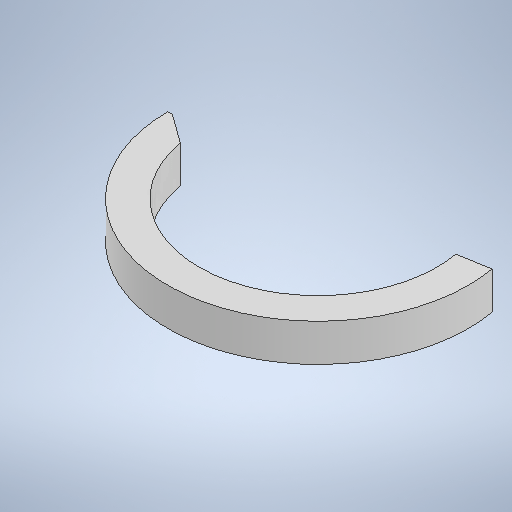
# Autodesk Inventor part: InertiaKitOuter
Saved by Autodesk Inventor 2025 (Build 290162000, 162)
## iProperties
Created: 2026-01-08
Part Number: InertiaKitOuter
Material: Generic
Document SubType Name: Modeling
Designer: tapen
Density: 1 g/cm^3
Appearance: Default
Author: tapen
Autodesk Inventor part; units mm, degrees
ref_plane "YZ Plane" through (0, 0, 0) normal (1, 0, 0) x (0, 1, 0)
ref_plane "XZ Plane" through (0, 0, 0) normal (0, 1, 0) x (-1, 0, 0)
ref_plane "XY Plane" through (0, 0, 0) normal (0, 0, 1) x (1, 0, 0)
sketch "Sketch1" plane through (0, 0, 0) normal (0, 0, 1) x (1, 0, 0)
  line L0 (-15, 0) -> (-15, 20)
  line L1 (-13, 22) -> (-2, 22)
  line L2 (0, 20) -> (0, 0)
  line L3 (0, 0) -> (3, 0)
  line L4 (3, 0) -> (3, 25)
  line L5 (3, 25) -> (-18, 25)
  line L6 (-18, 25) -> (-18, 0)
  line L7 (-18, 0) -> (-15, 0)
  line L8 (82.5, 0) -> (82.5, 23.5159) construction
  arc A0 (0, 20) -> (-2, 22) centre (-2, 20) ccw
  arc A1 (-13, 22) -> (-15, 20) centre (-13, 20) ccw
  point P0 (-15, 22)
  point P1 (0, 22)
  point P2 (-7.5, 0)
  dimension "d0" = 22
  dimension "d2" = 15
  dimension "d3" = 3
  dimension "d4" = 25
  dimension "d5" = 21
  dimension "d6" = 7.5
  dimension "d7" = 0
  dimension "d8" = 90
  dimension "d9" = 2
  dimension "d15" = 0
  constraints: 18 end point, 6 perpendicular, 4 point on circle, 4 point on line, 4 tangent, 2 centre point, 2 vertical, 1 equal radius, 1 horizontal
  measures "d0" distance of L0.start point (-15, 22)
  measures "d2" distance of point (-15, 22) point (0, 22)
  measures "d3" distance of L2.end L3.end
  measures "d4" distance of L3.end L4.end
  measures "d5" distance of L4.end L5.end
  measures "d6" distance from line of point (-7.5, 0) L2
  measures "d7" vertical distance of L2.end point (-7.5, 0)
  measures "d8" distance of L8.start point (-7.5, 0)
  measures "d9" radius of A0
  measures "d15" distance from line of L2.end L7
revolve "Revolution1" add sketch "Sketch1" angle 190 about axis through (82.5, 0, 0) along (0, 1, 0)
sketch "Sketch2" plane through (-18, 25, 0) normal (0, 1, 0) x (1, 0, 0)
  arc A0 (21, 0) -> (178.7922, 13.805) centre (100.5, 0) ccw projected
  arc A1 (3, 0) -> (196.5188, 16.9307) centre (100.5, 0) ccw projected
  line L0 (100.5, 0) -> (3, 0)
  line L1 (5, 0) -> (16, 0) projected
  line L2 (100.5, 0) -> (22.2078, -13.805)
  line L3 (22.2078, -13.805) -> (3, 0)
  point P0 (18, 0)
  point P1 (21, 0)
  dimension "d12" = 10
  constraints: 6 end point, 1 collinear, 1 point on circle
  measures "d12" angle of L0 L2
extrude "Extrusion1" cut sketch "Sketch2" against normal up to surface (25 mm away) contours A0 L3 L0
equation "\"d6\" = 0.5 * d2"
body "Solid1"
